Autodesk Fusion 360 part; units mm, degrees
(part 2 of 2)
sketch "Sketch37" plane through (0, 34, 0) normal (0, -1, 0) x (1, 0, 0)
  line L0 (112, 0) -> (98, 0)
  line L1 (98, 0) -> (98, -4.6)
  line L2 (98, -4.6) -> (112, -4.6)
  line L3 (112, -4.6) -> (112, 0)
  line L4 (105, 0) -> (105, -2.1)
  line L5 (107, -2.8) -> (103, -2.8)
  line L6 (103, -2.8) -> (103, -1.4)
  line L7 (103, -1.4) -> (107, -1.4)
  line L8 (107, -1.4) -> (107, -2.8)
  line L9 (107, -2.8) -> (103, -1.4) construction
  line L10 (103, -2.8) -> (107, -1.4) construction
  point P0 (105, -2.1)
  dimension "d205" = 2.1
  dimension "d206" = 4
  dimension "d207" = 1.4
  constraint midpoint L0 L4.start
  constraint perpendicular L0 L4
  constraint horizontal L5
  constraint perpendicular L5 L6
  constraint parallel L5 L7
  constraint parallel L6 L8
  constraint coincident L9 P0
  constraint coincident L10 P0
  constraint coincident P0 L4.end
  measures "d205" distance of L4.start P0
  measures "d206" distance of L6.end L7.end
  measures "d207" distance of L5.end L6.end
extrude "Extrude38" cut sketch "Sketch37" against normal blind 1 contours L5 L6 L7 L8
sketch "Sketch38" plane through (0, 50, 0) normal (0, -1, 0) x (1, 0, 0)
  line L0 (141, 0) -> (127, 0)
  line L1 (127, 0) -> (127, -4.6)
  line L2 (127, -4.6) -> (141, -4.6)
  line L3 (141, -4.6) -> (141, 0)
  line L4 (134, 0) -> (134, -2.1)
  line L5 (136, -2.8) -> (132, -2.8)
  line L6 (132, -2.8) -> (132, -1.4)
  line L7 (132, -1.4) -> (136, -1.4)
  line L8 (136, -1.4) -> (136, -2.8)
  line L9 (136, -2.8) -> (132, -1.4) construction
  line L10 (132, -2.8) -> (136, -1.4) construction
  point P0 (134, -2.1)
  dimension "d210" = 2.1
  dimension "d211" = 4
  dimension "d212" = 1.4
  constraint midpoint L0 L4.start
  constraint perpendicular L0 L4
  constraint horizontal L5
  constraint perpendicular L5 L6
  constraint parallel L5 L7
  constraint parallel L6 L8
  constraint coincident L9 P0
  constraint coincident L10 P0
  constraint coincident P0 L4.end
  measures "d210" distance of L4.start P0
  measures "d211" distance of L6.end L7.end
  measures "d212" distance of L5.end L6.end
extrude "Extrude39" cut sketch "Sketch38" against normal blind 1 contours L5 L6 L7 L8
sketch "Sketch39" plane through (0, 36, 0) normal (0, 1, 0) x (-1, 0, 0)
  line L0 (-127, 0) -> (-141, 0)
  line L1 (-141, 0) -> (-141, -4.6)
  line L2 (-141, -4.6) -> (-127, -4.6)
  line L3 (-127, -4.6) -> (-127, 0)
  line L4 (-134, 0) -> (-134, -2.1)
  line L5 (-132, -2.8) -> (-136, -2.8)
  line L6 (-136, -2.8) -> (-136, -1.4)
  line L7 (-136, -1.4) -> (-132, -1.4)
  line L8 (-132, -1.4) -> (-132, -2.8)
  line L9 (-132, -2.8) -> (-136, -1.4) construction
  line L10 (-136, -2.8) -> (-132, -1.4) construction
  point P0 (-134, -2.1)
  dimension "d215" = 2.1
  dimension "d216" = 4
  dimension "d217" = 1.4
  constraint midpoint L0 L4.start
  constraint perpendicular L0 L4
  constraint horizontal L5
  constraint perpendicular L5 L6
  constraint parallel L5 L7
  constraint parallel L6 L8
  constraint coincident L9 P0
  constraint coincident L10 P0
  constraint coincident P0 L4.end
  measures "d215" distance of L4.start P0
  measures "d216" distance of L6.end L7.end
  measures "d217" distance of L5.end L6.end
extrude "Extrude40" cut sketch "Sketch39" against normal blind 1 contours L5 L6 L7 L8
sketch "Sketch40" plane through (0, 17, 0) normal (0, 1, 0) x (-1, 0, 0)
  line L0 (-127, 0) -> (-141, 0)
  line L1 (-141, 0) -> (-141, -4.6)
  line L2 (-141, -4.6) -> (-127, -4.6)
  line L3 (-127, -4.6) -> (-127, 0)
  line L4 (-134, 0) -> (-134, -2.1)
  line L5 (-132, -2.8) -> (-136, -2.8)
  line L6 (-136, -2.8) -> (-136, -1.4)
  line L7 (-136, -1.4) -> (-132, -1.4)
  line L8 (-132, -1.4) -> (-132, -2.8)
  line L9 (-132, -2.8) -> (-136, -1.4) construction
  line L10 (-136, -2.8) -> (-132, -1.4) construction
  point P0 (-134, -2.1)
  dimension "d220" = 2.1
  dimension "d221" = 4
  dimension "d222" = 1.4
  constraint midpoint L0 L4.start
  constraint perpendicular L0 L4
  constraint horizontal L5
  constraint perpendicular L5 L6
  constraint parallel L5 L7
  constraint parallel L6 L8
  constraint coincident L9 P0
  constraint coincident L10 P0
  constraint coincident P0 L4.end
  measures "d220" distance of L4.start P0
  measures "d221" distance of L6.end L7.end
  measures "d222" distance of L5.end L6.end
extrude "Extrude41" cut sketch "Sketch40" against normal blind 1 contours L5 L6 L7 L8
sketch "Sketch41" plane through (0, 31, 0) normal (0, -1, 0) x (1, 0, 0)
  line L0 (141, 0) -> (127, 0)
  line L1 (127, 0) -> (127, -4.6)
  line L2 (127, -4.6) -> (141, -4.6)
  line L3 (141, -4.6) -> (141, 0)
  line L4 (134, 0) -> (134, -2.1)
  line L5 (136, -2.8) -> (132, -2.8)
  line L6 (132, -2.8) -> (132, -1.4)
  line L7 (132, -1.4) -> (136, -1.4)
  line L8 (136, -1.4) -> (136, -2.8)
  line L9 (136, -2.8) -> (132, -1.4) construction
  line L10 (132, -2.8) -> (136, -1.4) construction
  point P0 (134, -2.1)
  dimension "d225" = 2.1
  dimension "d226" = 4
  dimension "d227" = 1.4
  constraint midpoint L0 L4.start
  constraint perpendicular L0 L4
  constraint horizontal L5
  constraint perpendicular L5 L6
  constraint parallel L5 L7
  constraint parallel L6 L8
  constraint coincident L9 P0
  constraint coincident L10 P0
  constraint coincident P0 L4.end
  measures "d225" distance of L4.start P0
  measures "d226" distance of L6.end L7.end
  measures "d227" distance of L5.end L6.end
extrude "Extrude42" cut sketch "Sketch41" against normal blind 1 contours L5 L6 L7 L8
sketch "Sketch42" plane through (0, 34, 0) normal (0, -1, 0) x (1, 0, 0)
  line L0 (167, 0) -> (153, 0)
  line L1 (153, 0) -> (153, -4.6)
  line L2 (153, -4.6) -> (167, -4.6)
  line L3 (167, -4.6) -> (167, 0)
  line L4 (160, 0) -> (160, -2.1)
  line L5 (162, -2.8) -> (158, -2.8)
  line L6 (158, -2.8) -> (158, -1.4)
  line L7 (158, -1.4) -> (162, -1.4)
  line L8 (162, -1.4) -> (162, -2.8)
  line L9 (162, -2.8) -> (158, -1.4) construction
  line L10 (158, -2.8) -> (162, -1.4) construction
  point P0 (160, -2.1)
  dimension "d230" = 2.1
  dimension "d231" = 4
  dimension "d232" = 1.4
  constraint midpoint L0 L4.start
  constraint perpendicular L0 L4
  constraint horizontal L5
  constraint perpendicular L5 L6
  constraint parallel L5 L7
  constraint parallel L6 L8
  constraint coincident L9 P0
  constraint coincident L10 P0
  constraint coincident P0 L4.end
  measures "d230" distance of L4.start P0
  measures "d231" distance of L6.end L7.end
  measures "d232" distance of L5.end L6.end
extrude "Extrude43" cut sketch "Sketch42" against normal blind 1 contours L5 L6 L7 L8
sketch "Sketch43" plane through (0, 20, 0) normal (0, 1, 0) x (-1, 0, 0)
  line L0 (-153, 0) -> (-167, 0)
  line L1 (-167, 0) -> (-167, -4.6)
  line L2 (-167, -4.6) -> (-153, -4.6)
  line L3 (-153, -4.6) -> (-153, 0)
  line L4 (-160, 0) -> (-160, -2.1)
  line L5 (-158, -2.8) -> (-162, -2.8)
  line L6 (-162, -2.8) -> (-162, -1.4)
  line L7 (-162, -1.4) -> (-158, -1.4)
  line L8 (-158, -1.4) -> (-158, -2.8)
  line L9 (-158, -2.8) -> (-162, -1.4) construction
  line L10 (-162, -2.8) -> (-158, -1.4) construction
  point P0 (-160, -2.1)
  dimension "d235" = 2.1
  dimension "d236" = 4
  dimension "d237" = 1.4
  constraint midpoint L0 L4.start
  constraint perpendicular L0 L4
  constraint horizontal L5
  constraint perpendicular L5 L6
  constraint parallel L5 L7
  constraint parallel L6 L8
  constraint coincident L9 P0
  constraint coincident L10 P0
  constraint coincident P0 L4.end
  measures "d235" distance of L4.start P0
  measures "d236" distance of L6.end L7.end
  measures "d237" distance of L5.end L6.end
extrude "Extrude44" cut sketch "Sketch43" against normal blind 1 contours L5 L6 L7 L8
sketch "Sketch44" plane through (0, 1, 0) normal (0, 1, 0) x (-1, 0, 0)
  line L0 (-153, 0) -> (-167, 0)
  line L1 (-167, 0) -> (-167, -4.6)
  line L2 (-167, -4.6) -> (-153, -4.6)
  line L3 (-153, -4.6) -> (-153, 0)
  line L4 (-160, 0) -> (-160, -2.1)
  line L5 (-158, -2.8) -> (-162, -2.8)
  line L6 (-162, -2.8) -> (-162, -1.4)
  line L7 (-162, -1.4) -> (-158, -1.4)
  line L8 (-158, -1.4) -> (-158, -2.8)
  line L9 (-158, -2.8) -> (-162, -1.4) construction
  line L10 (-162, -2.8) -> (-158, -1.4) construction
  point P0 (-160, -2.1)
  dimension "d240" = 2.1
  dimension "d241" = 4
  dimension "d242" = 1.4
  constraint midpoint L0 L4.start
  constraint perpendicular L0 L4
  constraint horizontal L5
  constraint perpendicular L5 L6
  constraint parallel L5 L7
  constraint parallel L6 L8
  constraint coincident L9 P0
  constraint coincident L10 P0
  constraint coincident P0 L4.end
  measures "d240" distance of L4.start P0
  measures "d241" distance of L6.end L7.end
  measures "d242" distance of L5.end L6.end
extrude "Extrude45" cut sketch "Sketch44" against normal blind 1 contours L5 L6 L7 L8
sketch "Sketch45" plane through (0, 15, 0) normal (0, -1, 0) x (1, 0, 0)
  line L0 (167, 0) -> (153, 0)
  line L1 (153, 0) -> (153, -4.6)
  line L2 (153, -4.6) -> (167, -4.6)
  line L3 (167, -4.6) -> (167, 0)
  line L4 (160, 0) -> (160, -2.1)
  line L5 (162, -2.8) -> (158, -2.8)
  line L6 (158, -2.8) -> (158, -1.4)
  line L7 (158, -1.4) -> (162, -1.4)
  line L8 (162, -1.4) -> (162, -2.8)
  line L9 (162, -2.8) -> (158, -1.4) construction
  line L10 (158, -2.8) -> (162, -1.4) construction
  point P0 (160, -2.1)
  dimension "d245" = 2.1
  dimension "d246" = 4
  dimension "d247" = 1.4
  constraint midpoint L0 L4.start
  constraint perpendicular L0 L4
  constraint horizontal L5
  constraint perpendicular L5 L6
  constraint parallel L5 L7
  constraint parallel L6 L8
  constraint coincident L9 P0
  constraint coincident L10 P0
  constraint coincident P0 L4.end
  measures "d245" distance of L4.start P0
  measures "d246" distance of L6.end L7.end
  measures "d247" distance of L5.end L6.end
extrude "Extrude46" cut sketch "Sketch45" against normal blind 1 contours L5 L6 L7 L8
fillet "Fillet1" radius 1 8 edges at (-180.364, -66.364, 0) (-183, 0, 0) (-180.364, 66.364, 0) (0, 69, 0) (180.364, 66.364, 0) (183, 0, 0) (180.364, -66.364, 0) (0, -69, 0)
chamfer "Chamfer1" distance 0.4 angle 45 7 edges at (-170.5759, 58.0598, 0) (-170.5759, -59.9402, 0) (2.4241, -59.9402, 0) (-55.4241, 59.9402, 0) (50.5759, 59.9402, 0) (175.4241, -59.9402, 0) (175.4241, 58.0598, 0)
